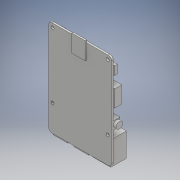
# Autodesk Inventor part: raspberry-pi-3-model
Saved by Autodesk Inventor 2018 (Build 220112000, 112)
## iProperties
Created: 2018-01-02
Part Number: raspberry-pi-3-model
Material: Generic
Document SubType Name: Modeling
Designer: rwradema
Density: 1 g/cm^3
Appearance: Default
Author: rwradema
Autodesk Inventor part; units mm, degrees
ref_plane "YZ Plane" through (0, 0, 0) normal (1, 0, 0) x (0, 1, 0)
ref_plane "XZ Plane" through (0, 0, 0) normal (0, 1, 0) x (-1, 0, 0)
ref_plane "XY Plane" through (0, 0, 0) normal (0, 0, 1) x (1, 0, 0)
sketch "Sketch1" plane through (0, 0, 0) normal (0, 1, 0) x (-1, 0, 0)
  line L0 (25, 42.5) -> (-25, 42.5)
  line L1 (-28, 39.5) -> (-28, -39.5)
  line L2 (-25, -42.5) -> (25, -42.5)
  line L3 (28, -39.5) -> (28, 39.5)
  line L4 (28, 42.5) -> (-28, -42.5) construction
  line L5 (-28, 42.5) -> (28, -42.5) construction
  arc A0 (28, 39.5) -> (25, 42.5) centre (25, 39.5) ccw
  arc A1 (-25, 42.5) -> (-28, 39.5) centre (-25, 39.5) ccw
  arc A2 (-28, -39.5) -> (-25, -42.5) centre (-25, -39.5) ccw
  arc A3 (25, -42.5) -> (28, -39.5) centre (25, -39.5) ccw
  point P0 (0, 0)
  dimension "d0" = 3
  dimension "d1" = 56
  dimension "d2" = 85
  constraints: 12 end point, 8 point on circle, 8 point on line, 8 tangent, 4 centre point, 3 equal radius, 2 midpoint, 2 parallel, 1 horizontal, 1 perpendicular
  measures "d0" radius of A0
  measures "d1" distance of L1.start L3.end
  measures "d2" distance between parallel lines of L2 L0
extrude "Extrusion1" add sketch "Sketch1" along normal blind 1.5748
sketch "Sketch2" plane through (0, 1.5748, 0) normal (0, 1, 0) x (1, 0, 0)
  circle A0 centre (-24.5, -39) radius 1.375
  circle A1 centre (24.5, -39) radius 1.375
  circle A2 centre (24.5, 19) radius 1.375
  circle A3 centre (-24.5, 19) radius 1.375
  line L0 (-25, -42.5) -> (25, -42.5) projected
  line L1 (-28, 39.5) -> (-28, -39.5) projected
  line L2 (28, -39.5) -> (28, 39.5) projected
  point P0 (0, 0)
  dimension "d5" = 2.75
  dimension "d6" = 3.5
  dimension "d7" = 3.5
  dimension "d8" = 58
  dimension "d9" = 3.5
  dimension "d10" = 3.5
  dimension "d11" = 3.5
  dimension "d12" = 3.5
  dimension "d13" = 58
  constraints: 4 centre point, 3 equal radius
  measures "d5" diameter of A0
  measures "d6" distance from line of L0 A0.centre
  measures "d7" distance from line of L1 A0.centre
  measures "d8" distance of A0.centre A3.centre
  measures "d9" distance from line of L0 A1.centre
  measures "d10" distance from line of L2 A1.centre
  measures "d11" distance from line of L2 A2.centre
  measures "d12" distance from line of L1 A3.centre
  measures "d13" distance of A1.centre A2.centre
extrude "Extrusion2" cut sketch "Sketch2" against normal up to next
sketch "Sketch3" plane through (0, 1.5748, 0) normal (0, 1, 0) x (1, 0, 0)
  line L0 (9.75, 23.15) -> (25.75, 23.15)
  line L1 (25.75, 23.15) -> (25.75, 44.35)
  line L2 (25.75, 44.35) -> (9.75, 44.35)
  line L3 (9.75, 44.35) -> (9.75, 23.15)
  line L4 (9.75, 23.15) -> (25.75, 44.35) construction
  line L5 (25.75, 23.15) -> (9.75, 44.35) construction
  line L6 (28, -39.5) -> (28, 39.5) projected
  line L7 (25, 42.5) -> (-25, 42.5) projected
  point P0 (0, 0)
  point P1 (17.75, 33.75)
  dimension "d16" = 21.2
  dimension "d17" = 16
  dimension "d18" = 10.25
  dimension "d19" = 1.85
  constraints: 12 end point, 2 midpoint, 2 parallel, 1 horizontal, 1 perpendicular
  measures "d16" distance of L2.end L0.start
  measures "d17" distance of L0.start L0.end
  measures "d18" distance from line of L6 point (17.75, 33.75)
  measures "d19" distance between parallel lines of L7 L2
extrude "Extrusion3" add sketch "Sketch3" along normal blind 13.82
sketch "Sketch4" plane through (0, 1.5748, 0) normal (0, 1, 0) x (1, 0, 0)
  line L0 (-25.5, 27.19) -> (-12.34, 27.19)
  line L1 (-12.34, 27.19) -> (-12.34, 44.84)
  line L2 (-12.34, 44.84) -> (-25.5, 44.84)
  line L3 (-25.5, 44.84) -> (-25.5, 27.19)
  line L4 (-7, 27.19) -> (6.16, 27.19)
  line L5 (6.16, 27.19) -> (6.16, 44.84)
  line L6 (6.16, 44.84) -> (-7, 44.84)
  line L7 (-7, 44.84) -> (-7, 27.19)
  line L8 (9.75, 42.5) -> (-25, 42.5) projected
  line L9 (28, -39.5) -> (28, 39.5) projected
  line L10 (-28, 39.5) -> (-28, -39.5) projected
  point P0 (0, 0)
  dimension "d22" = 13.16
  dimension "d23" = 17.65
  dimension "d24" = 2.34
  dimension "d25" = 35
  dimension "d26" = 2.5
  constraints: 16 end point, 4 parallel, 2 equal length, 2 horizontal, 2 perpendicular, 1 collinear
  measures "d22" distance of L0.start L0.end
  measures "d23" distance of L2.end L0.start
  measures "d24" distance between parallel lines of L8 L2
  measures "d25" distance between parallel lines of L9 L7
  measures "d26" distance between parallel lines of L3 L10
extrude "Extrusion4" add sketch "Sketch4" along normal blind 15
sketch "Sketch5" plane through (0, 1.5748, 0) normal (0, 1, 0) x (1, 0, 0)
  line L0 (-27.04, -35.4) -> (-21.96, -35.4) construction
  line L1 (-21.96, -35.4) -> (-21.96, 15.4) construction
  line L2 (-21.96, 15.4) -> (-27.04, 15.4) construction
  line L3 (-27.04, 15.4) -> (-27.04, -35.4) construction
  line L4 (-27.04, -35.4) -> (-21.96, 15.4) construction
  line L5 (-21.96, -35.4) -> (-27.04, 15.4) construction
  line L6 (-25, -42.5) -> (25, -42.5) construction
  line L7 (-28, 39.5) -> (-28, -39.5) construction
  circle A0 centre (-24.5, -39) radius 1.375 construction
  line L8 (-27.04, -35.4) -> (-21.96, -35.4)
  line L9 (-21.96, -35.4) -> (-21.96, 15.4)
  line L10 (-21.96, 15.4) -> (-27.04, 15.4)
  line L11 (-27.04, 15.4) -> (-27.04, -35.4)
  point P0 (0, 0)
  point P1 (-24.5, -10)
  dimension "d30" = 3.5
  dimension "d31" = 50.8
  dimension "d32" = 5.08
  dimension "d33" = 29
  constraints: 20 end point, 4 parallel, 2 horizontal, 2 midpoint, 2 perpendicular
  measures "d30" distance from line of L7 point (-24.5, -10)
  measures "d31" distance of L2.end L0.start
  measures "d32" distance of L0.start L0.end
  measures "d33" distance of point (-24.5, -10) A0.centre
extrude "Extrusion5" add sketch "Sketch5" along normal blind 2.54
sketch "Sketch6" plane through (0, 4.1148, 0) normal (0, 1, 0) x (1, 0, 0)
  line L0 (-25.98, -34.34) -> (-25.33, -34.34)
  line L1 (-25.33, -34.34) -> (-25.33, -33.69)
  line L2 (-25.33, -33.69) -> (-25.98, -33.69)
  line L3 (-25.98, -33.69) -> (-25.98, -34.34)
  line L4 (-27.04, 15.4) -> (-27.04, -35.4) projected
  line L5 (-27.04, -35.4) -> (-21.96, -35.4) projected
  line L6 (-25.98, -31.8) -> (-25.33, -31.8)
  line L7 (-25.33, -31.8) -> (-25.33, -31.15)
  line L8 (-25.33, -31.15) -> (-25.98, -31.15)
  line L9 (-25.98, -31.15) -> (-25.98, -31.8)
  line L10 (-25.98, -29.26) -> (-25.33, -29.26)
  line L11 (-25.33, -29.26) -> (-25.33, -28.61)
  line L12 (-25.33, -28.61) -> (-25.98, -28.61)
  line L13 (-25.98, -28.61) -> (-25.98, -29.26)
  line L14 (-25.98, -26.72) -> (-25.33, -26.72)
  line L15 (-25.33, -26.72) -> (-25.33, -26.07)
  line L16 (-25.33, -26.07) -> (-25.98, -26.07)
  line L17 (-25.98, -26.07) -> (-25.98, -26.72)
  line L18 (-25.98, -24.18) -> (-25.33, -24.18)
  line L19 (-25.33, -24.18) -> (-25.33, -23.53)
  line L20 (-25.33, -23.53) -> (-25.98, -23.53)
  line L21 (-25.98, -23.53) -> (-25.98, -24.18)
  line L22 (-25.98, -21.64) -> (-25.33, -21.64)
  line L23 (-25.33, -21.64) -> (-25.33, -20.99)
  line L24 (-25.33, -20.99) -> (-25.98, -20.99)
  line L25 (-25.98, -20.99) -> (-25.98, -21.64)
  line L26 (-25.98, -19.1) -> (-25.33, -19.1)
  line L27 (-25.33, -19.1) -> (-25.33, -18.45)
  line L28 (-25.33, -18.45) -> (-25.98, -18.45)
  line L29 (-25.98, -18.45) -> (-25.98, -19.1)
  line L30 (-25.98, -16.56) -> (-25.33, -16.56)
  line L31 (-25.33, -16.56) -> (-25.33, -15.91)
  line L32 (-25.33, -15.91) -> (-25.98, -15.91)
  line L33 (-25.98, -15.91) -> (-25.98, -16.56)
  line L34 (-25.98, -14.02) -> (-25.33, -14.02)
  line L35 (-25.33, -14.02) -> (-25.33, -13.37)
  line L36 (-25.33, -13.37) -> (-25.98, -13.37)
  line L37 (-25.98, -13.37) -> (-25.98, -14.02)
  line L38 (-25.98, -11.48) -> (-25.33, -11.48)
  line L39 (-25.33, -11.48) -> (-25.33, -10.83)
  line L40 (-25.33, -10.83) -> (-25.98, -10.83)
  line L41 (-25.98, -10.83) -> (-25.98, -11.48)
  line L42 (-25.98, -8.94) -> (-25.33, -8.94)
  line L43 (-25.33, -8.94) -> (-25.33, -8.29)
  line L44 (-25.33, -8.29) -> (-25.98, -8.29)
  line L45 (-25.98, -8.29) -> (-25.98, -8.94)
  line L46 (-25.98, -6.4) -> (-25.33, -6.4)
  line L47 (-25.33, -6.4) -> (-25.33, -5.75)
  line L48 (-25.33, -5.75) -> (-25.98, -5.75)
  line L49 (-25.98, -5.75) -> (-25.98, -6.4)
  line L50 (-25.98, -3.86) -> (-25.33, -3.86)
  line L51 (-25.33, -3.86) -> (-25.33, -3.21)
  line L52 (-25.33, -3.21) -> (-25.98, -3.21)
  line L53 (-25.98, -3.21) -> (-25.98, -3.86)
  line L54 (-25.98, -1.32) -> (-25.33, -1.32)
  line L55 (-25.33, -1.32) -> (-25.33, -0.67)
  line L56 (-25.33, -0.67) -> (-25.98, -0.67)
  line L57 (-25.98, -0.67) -> (-25.98, -1.32)
  line L58 (-25.98, 1.22) -> (-25.33, 1.22)
  line L59 (-25.33, 1.22) -> (-25.33, 1.87)
  line L60 (-25.33, 1.87) -> (-25.98, 1.87)
  line L61 (-25.98, 1.87) -> (-25.98, 1.22)
  line L62 (-25.98, 3.76) -> (-25.33, 3.76)
  line L63 (-25.33, 3.76) -> (-25.33, 4.41)
  line L64 (-25.33, 4.41) -> (-25.98, 4.41)
  line L65 (-25.98, 4.41) -> (-25.98, 3.76)
  line L66 (-25.98, 6.3) -> (-25.33, 6.3)
  line L67 (-25.33, 6.3) -> (-25.33, 6.95)
  line L68 (-25.33, 6.95) -> (-25.98, 6.95)
  line L69 (-25.98, 6.95) -> (-25.98, 6.3)
  line L70 (-25.98, 8.84) -> (-25.33, 8.84)
  line L71 (-25.33, 8.84) -> (-25.33, 9.49)
  line L72 (-25.33, 9.49) -> (-25.98, 9.49)
  line L73 (-25.98, 9.49) -> (-25.98, 8.84)
  line L74 (-25.98, 11.38) -> (-25.33, 11.38)
  line L75 (-25.33, 11.38) -> (-25.33, 12.03)
  line L76 (-25.33, 12.03) -> (-25.98, 12.03)
  line L77 (-25.98, 12.03) -> (-25.98, 11.38)
  line L78 (-25.98, 13.92) -> (-25.33, 13.92)
  line L79 (-25.33, 13.92) -> (-25.33, 14.57)
  line L80 (-25.33, 14.57) -> (-25.98, 14.57)
  line L81 (-25.98, 14.57) -> (-25.98, 13.92)
  line L82 (-23.44, -34.34) -> (-22.79, -34.34)
  line L83 (-22.79, -34.34) -> (-22.79, -33.69)
  line L84 (-22.79, -33.69) -> (-23.44, -33.69)
  line L85 (-23.44, -33.69) -> (-23.44, -34.34)
  line L86 (-23.44, -31.8) -> (-22.79, -31.8)
  line L87 (-22.79, -31.8) -> (-22.79, -31.15)
  line L88 (-22.79, -31.15) -> (-23.44, -31.15)
  line L89 (-23.44, -31.15) -> (-23.44, -31.8)
  line L90 (-23.44, -29.26) -> (-22.79, -29.26)
  line L91 (-22.79, -29.26) -> (-22.79, -28.61)
  line L92 (-22.79, -28.61) -> (-23.44, -28.61)
  line L93 (-23.44, -28.61) -> (-23.44, -29.26)
  line L94 (-23.44, -26.72) -> (-22.79, -26.72)
  line L95 (-22.79, -26.72) -> (-22.79, -26.07)
  line L96 (-22.79, -26.07) -> (-23.44, -26.07)
  line L97 (-23.44, -26.07) -> (-23.44, -26.72)
  line L98 (-23.44, -24.18) -> (-22.79, -24.18)
  line L99 (-22.79, -24.18) -> (-22.79, -23.53)
  line L100 (-22.79, -23.53) -> (-23.44, -23.53)
  line L101 (-23.44, -23.53) -> (-23.44, -24.18)
  line L102 (-23.44, -21.64) -> (-22.79, -21.64)
  line L103 (-22.79, -21.64) -> (-22.79, -20.99)
  line L104 (-22.79, -20.99) -> (-23.44, -20.99)
  line L105 (-23.44, -20.99) -> (-23.44, -21.64)
  line L106 (-23.44, -19.1) -> (-22.79, -19.1)
  line L107 (-22.79, -19.1) -> (-22.79, -18.45)
  line L108 (-22.79, -18.45) -> (-23.44, -18.45)
  line L109 (-23.44, -18.45) -> (-23.44, -19.1)
  line L110 (-23.44, -16.56) -> (-22.79, -16.56)
  line L111 (-22.79, -16.56) -> (-22.79, -15.91)
  line L112 (-22.79, -15.91) -> (-23.44, -15.91)
  line L113 (-23.44, -15.91) -> (-23.44, -16.56)
  line L114 (-23.44, -14.02) -> (-22.79, -14.02)
  line L115 (-22.79, -14.02) -> (-22.79, -13.37)
  line L116 (-22.79, -13.37) -> (-23.44, -13.37)
  line L117 (-23.44, -13.37) -> (-23.44, -14.02)
  line L118 (-23.44, -11.48) -> (-22.79, -11.48)
  line L119 (-22.79, -11.48) -> (-22.79, -10.83)
  line L120 (-22.79, -10.83) -> (-23.44, -10.83)
  line L121 (-23.44, -10.83) -> (-23.44, -11.48)
  line L122 (-23.44, -8.94) -> (-22.79, -8.94)
  line L123 (-22.79, -8.94) -> (-22.79, -8.29)
  line L124 (-22.79, -8.29) -> (-23.44, -8.29)
  line L125 (-23.44, -8.29) -> (-23.44, -8.94)
  line L126 (-23.44, -6.4) -> (-22.79, -6.4)
  line L127 (-22.79, -6.4) -> (-22.79, -5.75)
  line L128 (-22.79, -5.75) -> (-23.44, -5.75)
  line L129 (-23.44, -5.75) -> (-23.44, -6.4)
  line L130 (-23.44, -3.86) -> (-22.79, -3.86)
  line L131 (-22.79, -3.86) -> (-22.79, -3.21)
  line L132 (-22.79, -3.21) -> (-23.44, -3.21)
  line L133 (-23.44, -3.21) -> (-23.44, -3.86)
  line L134 (-23.44, -1.32) -> (-22.79, -1.32)
  line L135 (-22.79, -1.32) -> (-22.79, -0.67)
  line L136 (-22.79, -0.67) -> (-23.44, -0.67)
  line L137 (-23.44, -0.67) -> (-23.44, -1.32)
  line L138 (-23.44, 1.22) -> (-22.79, 1.22)
  line L139 (-22.79, 1.22) -> (-22.79, 1.87)
  line L140 (-22.79, 1.87) -> (-23.44, 1.87)
  line L141 (-23.44, 1.87) -> (-23.44, 1.22)
  line L142 (-23.44, 3.76) -> (-22.79, 3.76)
  line L143 (-22.79, 3.76) -> (-22.79, 4.41)
  line L144 (-22.79, 4.41) -> (-23.44, 4.41)
  line L145 (-23.44, 4.41) -> (-23.44, 3.76)
  line L146 (-23.44, 6.3) -> (-22.79, 6.3)
  line L147 (-22.79, 6.3) -> (-22.79, 6.95)
  line L148 (-22.79, 6.95) -> (-23.44, 6.95)
  line L149 (-23.44, 6.95) -> (-23.44, 6.3)
  line L150 (-23.44, 8.84) -> (-22.79, 8.84)
  line L151 (-22.79, 8.84) -> (-22.79, 9.49)
  line L152 (-22.79, 9.49) -> (-23.44, 9.49)
  line L153 (-23.44, 9.49) -> (-23.44, 8.84)
  line L154 (-23.44, 11.38) -> (-22.79, 11.38)
  line L155 (-22.79, 11.38) -> (-22.79, 12.03)
  line L156 (-22.79, 12.03) -> (-23.44, 12.03)
  line L157 (-23.44, 12.03) -> (-23.44, 11.38)
  line L158 (-23.44, 13.92) -> (-22.79, 13.92)
  line L159 (-22.79, 13.92) -> (-22.79, 14.57)
  line L160 (-22.79, 14.57) -> (-23.44, 14.57)
  line L161 (-23.44, 14.57) -> (-23.44, 13.92)
  point P0 (0, 0)
  dimension "d36" = 0.65
  dimension "d37" = 1.71
  dimension "d38" = 1.71
  dimension "d41" = 2.54
  dimension "d44" = 2.54
  constraints: 320 end point, 2 horizontal, 2 parallel, 2 perpendicular, 1 vertical, 312 other
  measures "d36" distance of L2.end L0.start
  measures "d37" distance between parallel lines of L4 L1
  measures "d38" distance between parallel lines of L5 L2
  measures "d41" distance of L0.start L6.start
  measures "d44" distance of L0.start L82.start
extrude "Extrusion6" add sketch "Sketch6" along normal blind 5.92
sketch "Sketch7" plane through (25.75, 1.5748, -44.35) normal (0, 0, -1) x (-1, 0, 0)
  line L0 (16, 13.82) -> (0, 13.82) construction
  line L1 (8, 13.82) -> (8, 0) construction
  line L2 (50.75, 0) -> (0.75, 0) construction
  line L3 (14.2, 11.22) -> (1.8, 11.22)
  line L4 (1.8, 11.22) -> (1.8, 4)
  line L5 (1.8, 4) -> (4.9, 4)
  line L6 (4.9, 4) -> (4.9, 2.2)
  line L7 (4.9, 2.2) -> (11.1, 2.2)
  line L8 (11.1, 2.2) -> (11.1, 4)
  line L9 (11.1, 4) -> (14.2, 4)
  line L10 (14.2, 4) -> (14.2, 11.22)
  line L11 (16, 0) -> (16, 13.82) projected
  line L12 (0, 0) -> (0, 13.82) projected
  point P0 (25.75, -1.5748)
  dimension "d49" = 1.8
  dimension "d50" = 1.8
  dimension "d51" = 2.6
  dimension "d52" = 4
  dimension "d53" = 2.2
  dimension "d54" = 6.2
  constraints: 18 end point, 7 perpendicular, 3 point on line, 1 collinear, 1 midpoint, 1 vertical
  measures "d49" distance between parallel lines of L11 L10
  measures "d50" distance between parallel lines of L12 L4
  measures "d51" distance between parallel lines of L0 L3
  measures "d52" distance between parallel lines of L2 L5
  measures "d53" distance from line of L1.end L7
  measures "d54" distance of L6.end L7.end
extrude "Extrusion7" cut sketch "Sketch7" against normal blind 11.15
sketch "Sketch8" plane through (0, 1.5748, 0) normal (0, 1, 0) x (1, 0, 0)
  line L0 (23.6, -35.7) -> (29.2, -35.7)
  line L1 (29.2, -35.7) -> (29.2, -28.1)
  line L2 (29.2, -28.1) -> (23.6, -28.1)
  line L3 (23.6, -28.1) -> (23.6, -35.7)
  line L4 (23.6, -35.7) -> (29.2, -28.1) construction
  line L5 (29.2, -35.7) -> (23.6, -28.1) construction
  line L6 (-25, -42.5) -> (25, -42.5) projected
  line L7 (28, -39.5) -> (28, 39.5) projected
  point P0 (0, 0)
  point P1 (26.4, -31.9)
  dimension "d57" = 10.6
  dimension "d58" = 5.6
  dimension "d59" = 7.6
  dimension "d60" = 1.2
  constraints: 12 end point, 2 midpoint, 2 parallel, 1 horizontal, 1 perpendicular
  measures "d57" distance from line of L6 point (26.4, -31.9)
  measures "d58" distance of L1.end L2.end
  measures "d59" distance of L2.end L0.start
  measures "d60" distance between parallel lines of L7 L1
extrude "Extrusion8" add sketch "Sketch8" along normal blind 2.44
sketch "Sketch9" plane through (0, 1.5748, 0) normal (0, 1, 0) x (1, 0, 0)
  line L0 (18.25, -18) -> (29.25, -18)
  line L1 (29.25, -18) -> (29.25, -3)
  line L2 (29.25, -3) -> (18.25, -3)
  line L3 (18.25, -3) -> (18.25, -18)
  line L4 (18.25, -18) -> (29.25, -3) construction
  line L5 (29.25, -18) -> (18.25, -3) construction
  line L6 (-25, -42.5) -> (25, -42.5) projected
  line L7 (28, -28.1) -> (28, 39.5) projected
  point P0 (0, 0)
  point P1 (23.75, -10.5)
  dimension "d63" = 32
  dimension "d64" = 15
  dimension "d65" = 11
  dimension "d66" = 1.25
  constraints: 12 end point, 2 midpoint, 2 parallel, 1 horizontal, 1 perpendicular
  measures "d63" distance from line of L6 point (23.75, -10.5)
  measures "d64" distance of L2.end L0.start
  measures "d65" distance of L1.end L2.end
  measures "d66" distance between parallel lines of L7 L1
extrude "Extrusion9" add sketch "Sketch9" along normal blind 6.17
sketch "Sketch10" plane through (0, 1.5748, 0) normal (0, 1, 0) x (1, 0, 0)
  line L0 (15.5, 7.37) -> (28, 7.37)
  line L1 (28, 7.37) -> (28, 14.63)
  line L2 (28, 14.63) -> (15.5, 14.63)
  line L3 (15.5, 14.63) -> (15.5, 7.37)
  line L4 (15.5, 7.37) -> (28, 14.63) construction
  line L5 (28, 7.37) -> (15.5, 14.63) construction
  line L6 (-25, -42.5) -> (25, -42.5) projected
  line L7 (28, -3) -> (28, 39.5) projected
  point P0 (0, 0)
  point P1 (21.75, 11)
  dimension "d69" = 7.26
  dimension "d70" = 12.5
  dimension "d71" = 53.5
  constraints: 12 end point, 2 midpoint, 2 parallel, 1 collinear, 1 horizontal, 1 perpendicular
  measures "d69" distance of L2.end L0.start
  measures "d70" distance of L0.start L0.end
  measures "d71" distance from line of L6 point (21.75, 11)
extrude "Extrusion10" add sketch "Sketch10" along normal blind 5.84
sketch "Sketch11" plane through (28, 0, 39.5) normal (1, 0, 0) x (0, 0, -1)
  line L0 (46.87, 1.5748) -> (46.87, 7.4148) construction
  line L1 (46.87, 4.4948) -> (54.13, 4.4948) construction
  line L2 (54.13, 1.5748) -> (54.13, 7.4148) construction
  line L3 (46.87, 7.4148) -> (54.13, 7.4148) construction
  line L4 (50.5, 7.4148) -> (50.5, -4.4423) construction
  circle A0 centre (50.5, 4.4948) radius 2.95
  point P0 (39.5, 0)
  dimension "d74" = 5.9
  constraints: 4 end point, 4 midpoint, 1 centre point, 1 point on line, 1 vertical
  measures "d74" diameter of A0
extrude "Extrusion11" add sketch "Sketch11" along normal blind 2.46
sketch "Sketch12" plane through (0, 0, 0) normal (0, -1, 0) x (1, 0, 0)
  line L0 (6, 29.3) -> (-6, 29.3)
  line L1 (-6, 29.3) -> (-6, 44.8)
  line L2 (-6, 44.8) -> (6, 44.8)
  line L3 (6, 44.8) -> (6, 29.3)
  line L4 (6, 29.3) -> (-6, 44.8) construction
  line L5 (-6, 29.3) -> (6, 44.8) construction
  line L6 (-25, 42.5) -> (25, 42.5) projected
  line L7 (-28, -39.5) -> (-28, 39.5) projected
  point P0 (0, 0)
  point P1 (0, 37.05)
  dimension "d77" = 12
  dimension "d78" = 15.5
  dimension "d79" = 13.2
  dimension "d80" = 34
  constraints: 12 end point, 2 midpoint, 2 parallel, 1 horizontal, 1 perpendicular
  measures "d77" distance of L0.start L0.end
  measures "d78" distance of L0.end L1.end
  measures "d79" distance between parallel lines of L6 L0
  measures "d80" distance between parallel lines of L7 L3
extrude "Extrusion12" add sketch "Sketch12" along normal blind 1.4
body "Solid1"
